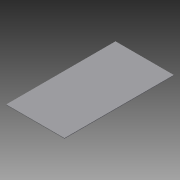
# Autodesk Inventor part: polycarb
Saved by Autodesk Inventor 2014 (Build 180170000, 170)
## iProperties
Created: 2013-09-21
Part Number: polycarb
Material: Generic
Document SubType Name: Modeling
Designer: Ryan
Density: 1 g/cm^3
Appearance: Default
Author: Ryan
Autodesk Inventor part; units mm, degrees
ref_plane "YZ Plane" through (0, 0, 0) normal (1, 0, 0) x (0, 1, 0)
ref_plane "XZ Plane" through (0, 0, 0) normal (0, 1, 0) x (-1, 0, 0)
ref_plane "XY Plane" through (0, 0, 0) normal (0, 0, 1) x (1, 0, 0)
sketch "Sketch1" plane through (0, 0, 0) normal (0, 1, 0) x (-1, 0, 0)
  line L0 (83.5914, -156.7307) -> (-83.5914, -156.7307)
  line L1 (-83.5914, -156.7307) -> (-83.5914, 156.7307)
  line L2 (-83.5914, 156.7307) -> (83.5914, 156.7307)
  line L3 (83.5914, 156.7307) -> (83.5914, -156.7307)
  line L4 (83.5914, -156.7307) -> (-83.5914, 156.7307) construction
  line L5 (-83.5914, -156.7307) -> (83.5914, 156.7307) construction
  point P0 (0, 0)
  dimension "d0" = 167.1828
  dimension "d1" = 313.4614
  constraints: 12 end point, 2 midpoint, 2 parallel, 1 horizontal, 1 perpendicular
  measures "d0" distance of L1.end L2.end
  measures "d1" distance of L0.end L1.end
extrude "Extrusion1" add sketch "Sketch1" along normal blind 1.5875
body "Solid1"
